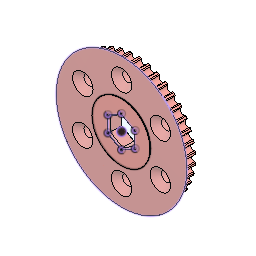
HTD Flanged Pulley Half (Autodesk Fusion 360 design; units mm, degrees)
Autodesk Fusion 360 part; units mm, degrees
sketch "Basic Outline" plane through (0, 0, 0) normal (0, 0, 1) x (1, 0, 0) in component "HTD 5M Pulley"
  circle A0 centre (0, 0) radius 31.2595
  line L0 (0, 0) -> (0, 30.7245) construction
  arc A1 (-1.5246, 30.758) -> (-1.9818, 31.1966) centre (-1.9545, 30.7675) ccw
  arc A2 (-1.5246, 30.758) -> (1.5246, 30.758) centre (0, 30.7245) ccw
  arc A3 (1.9818, 31.1966) -> (1.5246, 30.758) centre (1.9545, 30.7675) ccw
  dimension "d12" = 3.05
  dimension "d19" = 62.519
  dimension "d20" = 29.1995
  dimension "d21" = 0.43
  constraint coincident A0.centre L0.start
  constraint coincident L0.end A2.centre
  constraint tangent A1 A2
  constraint tangent A0 A1
  constraint coincident A0 A1.end
  constraint vertical L0
  constraint tangent A0 A3
  constraint tangent A2 A3
  constraint coincident A0 A3.start
  constraint equal A1 A3
  measures "d12" diameter of A2
  measures "d19" diameter of A0
  measures "d20" distance of A0.centre A2
  measures "d21" radius of A1
extrude "Extrude1" add sketch "Basic Outline" along normal blind 5.5 in component "HTD 5M Pulley"
extrude "Extrude2" cut sketch "Basic Outline" along normal blind 5.5 contours A0 A1 A2 A3 picked at (0, 30.5682) in component "HTD 5M Pulley"
pattern_circular "C-Pattern1" count 40 over 360 about axis through (0, 0, 1.75) along (0, 0, 1) of "Extrude2" in component "HTD 5M Pulley"
sketch "Flange" plane through (0, 0, 5.5) normal (0, 0, 1) x (1, 0, 0) in component "HTD 5M Pulley"
  arc A0 (6.8376, 30.5025) -> (6.3175, 30.1408) centre (6.7436, 30.0829) ccw
  arc A1 (3.3058, 30.6178) -> (6.3175, 30.1408) centre (4.8064, 30.3462) ccw
  arc A2 (3.3058, 30.6178) -> (2.9228, 31.1225) centre (2.8826, 30.6944) ccw
  arc A3 (2.9228, 31.1225) -> (1.9818, 31.1966) centre (0, 0) ccw
  arc A4 (1.9818, 31.1966) -> (1.5246, 30.758) centre (1.9545, 30.7675) ccw
  arc A5 (-1.5246, 30.758) -> (1.5246, 30.758) centre (0, 30.7245) ccw
  arc A6 (-1.5246, 30.758) -> (-1.9818, 31.1966) centre (-1.9545, 30.7675) ccw
  arc A7 (-1.9818, 31.1966) -> (-2.9228, 31.1225) centre (0, 0) ccw
  arc A8 (-2.9228, 31.1225) -> (-3.3058, 30.6178) centre (-2.8826, 30.6944) ccw
  arc A9 (-6.3175, 30.1408) -> (-3.3058, 30.6178) centre (-4.8064, 30.3462) ccw
  arc A10 (-6.3175, 30.1408) -> (-6.8376, 30.5025) centre (-6.7436, 30.0829) ccw
  arc A11 (-6.8376, 30.5025) -> (-7.7555, 30.2821) centre (0, 0) ccw
  arc A12 (-7.7555, 30.2821) -> (-8.0547, 29.7237) centre (-7.6488, 29.8656) ccw
  arc A13 (-10.9548, 28.7815) -> (-8.0547, 29.7237) centre (-9.4944, 29.2207) ccw
  arc A14 (-10.9548, 28.7815) -> (-11.5251, 29.0573) centre (-11.3665, 28.6576) ccw
  arc A15 (-11.5251, 29.0573) -> (-12.3972, 28.6961) centre (0, 0) ccw
  arc A16 (-12.3972, 28.6961) -> (-12.6054, 28.0978) centre (-12.2266, 28.3014) ccw
  arc A17 (-15.3223, 26.7134) -> (-12.6054, 28.0978) centre (-13.9486, 27.3757) ccw
  arc A18 (-15.3223, 26.7134) -> (-15.9287, 26.8967) centre (-15.7096, 26.5267) ccw
  arc A19 (-15.9287, 26.8967) -> (-16.7336, 26.4034) centre (0, 0) ccw
  arc A20 (-16.7336, 26.4034) -> (-16.8457, 25.7799) centre (-16.5034, 26.0402) ccw
  arc A21 (-19.3126, 23.9876) -> (-16.8457, 25.7799) centre (-18.0594, 24.8566) ccw
  arc A22 (-19.3126, 23.9876) -> (-19.9402, 24.0737) centre (-19.6659, 23.7426) ccw
  arc A23 (-19.9402, 24.0737) -> (-20.658, 23.4607) centre (0, 0) ccw
  arc A24 (-20.658, 23.4607) -> (-20.6711, 22.8273) centre (-20.3738, 23.1379) ccw
  arc A25 (-22.8273, 20.6711) -> (-20.6711, 22.8273) centre (-21.7255, 21.7255) ccw
  arc A26 (-22.8273, 20.6711) -> (-23.4607, 20.658) centre (-23.1379, 20.3738) ccw
  arc A27 (-23.4607, 20.658) -> (-24.0737, 19.9402) centre (0, 0) ccw
  arc A28 (-24.0737, 19.9402) -> (-23.9876, 19.3126) centre (-23.7426, 19.6659) ccw
  arc A29 (-25.7799, 16.8457) -> (-23.9876, 19.3126) centre (-24.8566, 18.0594) ccw
  arc A30 (-25.7799, 16.8457) -> (-26.4034, 16.7336) centre (-26.0402, 16.5034) ccw
  arc A31 (-26.4034, 16.7336) -> (-26.8967, 15.9287) centre (0, 0) ccw
  arc A32 (-26.8967, 15.9287) -> (-26.7134, 15.3223) centre (-26.5267, 15.7096) ccw
  arc A33 (-28.0978, 12.6054) -> (-26.7134, 15.3223) centre (-27.3757, 13.9486) ccw
  arc A34 (-28.0978, 12.6054) -> (-28.6961, 12.3972) centre (-28.3014, 12.2266) ccw
  arc A35 (-28.6961, 12.3972) -> (-29.0573, 11.5251) centre (0, 0) ccw
  arc A36 (-29.0573, 11.5251) -> (-28.7815, 10.9548) centre (-28.6576, 11.3665) ccw
  arc A37 (-29.7237, 8.0547) -> (-28.7815, 10.9548) centre (-29.2207, 9.4944) ccw
  arc A38 (-29.7237, 8.0547) -> (-30.2821, 7.7555) centre (-29.8656, 7.6488) ccw
  arc A39 (-30.2821, 7.7555) -> (-30.5025, 6.8376) centre (0, 0) ccw
  arc A40 (-30.5025, 6.8376) -> (-30.1408, 6.3175) centre (-30.0829, 6.7436) ccw
  arc A41 (-30.6178, 3.3058) -> (-30.1408, 6.3175) centre (-30.3462, 4.8064) ccw
  arc A42 (-30.6178, 3.3058) -> (-31.1225, 2.9228) centre (-30.6944, 2.8826) ccw
  arc A43 (-31.1225, 2.9228) -> (-31.1966, 1.9818) centre (0, 0) ccw
  arc A44 (-31.1966, 1.9818) -> (-30.758, 1.5246) centre (-30.7675, 1.9545) ccw
  arc A45 (-30.758, -1.5246) -> (-30.758, 1.5246) centre (-30.7245, 0) ccw
  arc A46 (-30.758, -1.5246) -> (-31.1966, -1.9818) centre (-30.7675, -1.9545) ccw
  arc A47 (-31.1966, -1.9818) -> (-31.1225, -2.9228) centre (0, 0) ccw
  arc A48 (-31.1225, -2.9228) -> (-30.6178, -3.3058) centre (-30.6944, -2.8826) ccw
  arc A49 (-30.1408, -6.3175) -> (-30.6178, -3.3058) centre (-30.3462, -4.8064) ccw
  arc A50 (-30.1408, -6.3175) -> (-30.5025, -6.8376) centre (-30.0829, -6.7436) ccw
  arc A51 (-30.5025, -6.8376) -> (-30.2821, -7.7555) centre (0, 0) ccw
  arc A52 (-30.2821, -7.7555) -> (-29.7237, -8.0547) centre (-29.8656, -7.6488) ccw
  arc A53 (-28.7815, -10.9548) -> (-29.7237, -8.0547) centre (-29.2207, -9.4944) ccw
  arc A54 (-28.7815, -10.9548) -> (-29.0573, -11.5251) centre (-28.6576, -11.3665) ccw
  arc A55 (-29.0573, -11.5251) -> (-28.6961, -12.3972) centre (0, 0) ccw
  arc A56 (-28.6961, -12.3972) -> (-28.0978, -12.6054) centre (-28.3014, -12.2266) ccw
  arc A57 (-26.7134, -15.3223) -> (-28.0978, -12.6054) centre (-27.3757, -13.9486) ccw
  arc A58 (-26.7134, -15.3223) -> (-26.8967, -15.9287) centre (-26.5267, -15.7096) ccw
  arc A59 (-26.8967, -15.9287) -> (-26.4034, -16.7336) centre (0, 0) ccw
  arc A60 (-26.4034, -16.7336) -> (-25.7799, -16.8457) centre (-26.0402, -16.5034) ccw
  arc A61 (-23.9876, -19.3126) -> (-25.7799, -16.8457) centre (-24.8566, -18.0594) ccw
  arc A62 (-23.9876, -19.3126) -> (-24.0737, -19.9402) centre (-23.7426, -19.6659) ccw
  arc A63 (-24.0737, -19.9402) -> (-23.4607, -20.658) centre (0, 0) ccw
  arc A64 (-23.4607, -20.658) -> (-22.8273, -20.6711) centre (-23.1379, -20.3738) ccw
  arc A65 (-20.6711, -22.8273) -> (-22.8273, -20.6711) centre (-21.7255, -21.7255) ccw
  arc A66 (-20.6711, -22.8273) -> (-20.658, -23.4607) centre (-20.3738, -23.1379) ccw
  arc A67 (-20.658, -23.4607) -> (-19.9402, -24.0737) centre (0, 0) ccw
  arc A68 (-19.9402, -24.0737) -> (-19.3126, -23.9876) centre (-19.6659, -23.7426) ccw
  arc A69 (-16.8457, -25.7799) -> (-19.3126, -23.9876) centre (-18.0594, -24.8566) ccw
  arc A70 (-16.8457, -25.7799) -> (-16.7336, -26.4034) centre (-16.5034, -26.0402) ccw
  arc A71 (-16.7336, -26.4034) -> (-15.9287, -26.8967) centre (0, 0) ccw
  arc A72 (-15.9287, -26.8967) -> (-15.3223, -26.7134) centre (-15.7096, -26.5267) ccw
  arc A73 (-12.6054, -28.0978) -> (-15.3223, -26.7134) centre (-13.9486, -27.3757) ccw
  arc A74 (-12.6054, -28.0978) -> (-12.3972, -28.6961) centre (-12.2266, -28.3014) ccw
  arc A75 (-12.3972, -28.6961) -> (-11.5251, -29.0573) centre (0, 0) ccw
  arc A76 (-11.5251, -29.0573) -> (-10.9548, -28.7815) centre (-11.3665, -28.6576) ccw
  arc A77 (-8.0547, -29.7237) -> (-10.9548, -28.7815) centre (-9.4944, -29.2207) ccw
  arc A78 (-8.0547, -29.7237) -> (-7.7555, -30.2821) centre (-7.6488, -29.8656) ccw
  arc A79 (-7.7555, -30.2821) -> (-6.8376, -30.5025) centre (0, 0) ccw
  arc A80 (-6.8376, -30.5025) -> (-6.3175, -30.1408) centre (-6.7436, -30.0829) ccw
  arc A81 (-3.3058, -30.6178) -> (-6.3175, -30.1408) centre (-4.8064, -30.3462) ccw
  arc A82 (-3.3058, -30.6178) -> (-2.9228, -31.1225) centre (-2.8826, -30.6944) ccw
  arc A83 (-2.9228, -31.1225) -> (-1.9818, -31.1966) centre (0, 0) ccw
  arc A84 (-1.9818, -31.1966) -> (-1.5246, -30.758) centre (-1.9545, -30.7675) ccw
  arc A85 (1.5246, -30.758) -> (-1.5246, -30.758) centre (0, -30.7245) ccw
  arc A86 (1.5246, -30.758) -> (1.9818, -31.1966) centre (1.9545, -30.7675) ccw
  arc A87 (1.9818, -31.1966) -> (2.9228, -31.1225) centre (0, 0) ccw
  arc A88 (2.9228, -31.1225) -> (3.3058, -30.6178) centre (2.8826, -30.6944) ccw
  arc A89 (6.3175, -30.1408) -> (3.3058, -30.6178) centre (4.8064, -30.3462) ccw
  arc A90 (6.3175, -30.1408) -> (6.8376, -30.5025) centre (6.7436, -30.0829) ccw
  arc A91 (6.8376, -30.5025) -> (7.7555, -30.2821) centre (0, 0) ccw
  arc A92 (7.7555, -30.2821) -> (8.0547, -29.7237) centre (7.6488, -29.8656) ccw
  arc A93 (10.9548, -28.7815) -> (8.0547, -29.7237) centre (9.4944, -29.2207) ccw
  arc A94 (10.9548, -28.7815) -> (11.5251, -29.0573) centre (11.3665, -28.6576) ccw
  arc A95 (11.5251, -29.0573) -> (12.3972, -28.6961) centre (0, 0) ccw
  arc A96 (12.3972, -28.6961) -> (12.6054, -28.0978) centre (12.2266, -28.3014) ccw
  arc A97 (15.3223, -26.7134) -> (12.6054, -28.0978) centre (13.9486, -27.3757) ccw
  arc A98 (15.3223, -26.7134) -> (15.9287, -26.8967) centre (15.7096, -26.5267) ccw
  arc A99 (15.9287, -26.8967) -> (16.7336, -26.4034) centre (0, 0) ccw
  arc A100 (16.7336, -26.4034) -> (16.8457, -25.7799) centre (16.5034, -26.0402) ccw
  arc A101 (19.3126, -23.9876) -> (16.8457, -25.7799) centre (18.0594, -24.8566) ccw
  arc A102 (19.3126, -23.9876) -> (19.9402, -24.0737) centre (19.6659, -23.7426) ccw
  arc A103 (19.9402, -24.0737) -> (20.658, -23.4607) centre (0, 0) ccw
  arc A104 (20.658, -23.4607) -> (20.6711, -22.8273) centre (20.3738, -23.1379) ccw
  arc A105 (22.8273, -20.6711) -> (20.6711, -22.8273) centre (21.7255, -21.7255) ccw
  arc A106 (22.8273, -20.6711) -> (23.4607, -20.658) centre (23.1379, -20.3738) ccw
  arc A107 (23.4607, -20.658) -> (24.0737, -19.9402) centre (0, 0) ccw
  arc A108 (24.0737, -19.9402) -> (23.9876, -19.3126) centre (23.7426, -19.6659) ccw
  arc A109 (25.7799, -16.8457) -> (23.9876, -19.3126) centre (24.8566, -18.0594) ccw
  arc A110 (25.7799, -16.8457) -> (26.4034, -16.7336) centre (26.0402, -16.5034) ccw
  arc A111 (26.4034, -16.7336) -> (26.8967, -15.9287) centre (0, 0) ccw
  arc A112 (26.8967, -15.9287) -> (26.7134, -15.3223) centre (26.5267, -15.7096) ccw
  arc A113 (28.0978, -12.6054) -> (26.7134, -15.3223) centre (27.3757, -13.9486) ccw
  arc A114 (28.0978, -12.6054) -> (28.6961, -12.3972) centre (28.3014, -12.2266) ccw
  arc A115 (28.6961, -12.3972) -> (29.0573, -11.5251) centre (0, 0) ccw
  arc A116 (29.0573, -11.5251) -> (28.7815, -10.9548) centre (28.6576, -11.3665) ccw
  arc A117 (29.7237, -8.0547) -> (28.7815, -10.9548) centre (29.2207, -9.4944) ccw
  arc A118 (29.7237, -8.0547) -> (30.2821, -7.7555) centre (29.8656, -7.6488) ccw
  arc A119 (30.2821, -7.7555) -> (30.5025, -6.8376) centre (0, 0) ccw
  arc A120 (30.5025, -6.8376) -> (30.1408, -6.3175) centre (30.0829, -6.7436) ccw
  arc A121 (30.6178, -3.3058) -> (30.1408, -6.3175) centre (30.3462, -4.8064) ccw
  arc A122 (30.6178, -3.3058) -> (31.1225, -2.9228) centre (30.6944, -2.8826) ccw
  arc A123 (31.1225, -2.9228) -> (31.1966, -1.9818) centre (0, 0) ccw
  arc A124 (31.1966, -1.9818) -> (30.758, -1.5246) centre (30.7675, -1.9545) ccw
  arc A125 (30.758, 1.5246) -> (30.758, -1.5246) centre (30.7245, 0) ccw
  arc A126 (30.758, 1.5246) -> (31.1966, 1.9818) centre (30.7675, 1.9545) ccw
  arc A127 (31.1966, 1.9818) -> (31.1225, 2.9228) centre (0, 0) ccw
  arc A128 (31.1225, 2.9228) -> (30.6178, 3.3058) centre (30.6944, 2.8826) ccw
  arc A129 (30.1408, 6.3175) -> (30.6178, 3.3058) centre (30.3462, 4.8064) ccw
  arc A130 (30.1408, 6.3175) -> (30.5025, 6.8376) centre (30.0829, 6.7436) ccw
  arc A131 (30.5025, 6.8376) -> (30.2821, 7.7555) centre (0, 0) ccw
  arc A132 (30.2821, 7.7555) -> (29.7237, 8.0547) centre (29.8656, 7.6488) ccw
  arc A133 (28.7815, 10.9548) -> (29.7237, 8.0547) centre (29.2207, 9.4944) ccw
  arc A134 (28.7815, 10.9548) -> (29.0573, 11.5251) centre (28.6576, 11.3665) ccw
  arc A135 (29.0573, 11.5251) -> (28.6961, 12.3972) centre (0, 0) ccw
  arc A136 (28.6961, 12.3972) -> (28.0978, 12.6054) centre (28.3014, 12.2266) ccw
  arc A137 (26.7134, 15.3223) -> (28.0978, 12.6054) centre (27.3757, 13.9486) ccw
  arc A138 (26.7134, 15.3223) -> (26.8967, 15.9287) centre (26.5267, 15.7096) ccw
  arc A139 (26.8967, 15.9287) -> (26.4034, 16.7336) centre (0, 0) ccw
  arc A140 (26.4034, 16.7336) -> (25.7799, 16.8457) centre (26.0402, 16.5034) ccw
  arc A141 (23.9876, 19.3126) -> (25.7799, 16.8457) centre (24.8566, 18.0594) ccw
  arc A142 (23.9876, 19.3126) -> (24.0737, 19.9402) centre (23.7426, 19.6659) ccw
  arc A143 (24.0737, 19.9402) -> (23.4607, 20.658) centre (0, 0) ccw
  arc A144 (23.4607, 20.658) -> (22.8273, 20.6711) centre (23.1379, 20.3738) ccw
  arc A145 (20.6711, 22.8273) -> (22.8273, 20.6711) centre (21.7255, 21.7255) ccw
  arc A146 (20.6711, 22.8273) -> (20.658, 23.4607) centre (20.3738, 23.1379) ccw
  arc A147 (20.658, 23.4607) -> (19.9402, 24.0737) centre (0, 0) ccw
  arc A148 (19.9402, 24.0737) -> (19.3126, 23.9876) centre (19.6659, 23.7426) ccw
  arc A149 (16.8457, 25.7799) -> (19.3126, 23.9876) centre (18.0594, 24.8566) ccw
  arc A150 (16.8457, 25.7799) -> (16.7336, 26.4034) centre (16.5034, 26.0402) ccw
  arc A151 (16.7336, 26.4034) -> (15.9287, 26.8967) centre (0, 0) ccw
  arc A152 (15.9287, 26.8967) -> (15.3223, 26.7134) centre (15.7096, 26.5267) ccw
  arc A153 (12.6054, 28.0978) -> (15.3223, 26.7134) centre (13.9486, 27.3757) ccw
  arc A154 (12.6054, 28.0978) -> (12.3972, 28.6961) centre (12.2266, 28.3014) ccw
  arc A155 (12.3972, 28.6961) -> (11.5251, 29.0573) centre (0, 0) ccw
  arc A156 (11.5251, 29.0573) -> (10.9548, 28.7815) centre (11.3665, 28.6576) ccw
  arc A157 (8.0547, 29.7237) -> (10.9548, 28.7815) centre (9.4944, 29.2207) ccw
  arc A158 (8.0547, 29.7237) -> (7.7555, 30.2821) centre (7.6488, 29.8656) ccw
  arc A159 (7.7555, 30.2821) -> (6.8376, 30.5025) centre (0, 0) ccw
  circle A160 centre (0, 0) radius 31.2595 construction
  circle A161 centre (0, 0) radius 33.7595
  circle A162 centre (0, 0) radius 83.7595
  dimension "d58" = 2.5
  dimension "d59" = 50
  constraint concentric A160 A161
  constraint concentric A3 A162
  measures "d58" distance of A160 A161
  measures "d59" distance of A161 A162
extrude "Extrude3" add sketch "Basic Outline" along normal blind 1.45 draft 60 from surface at 5.5 in component "HTD 5M Pulley"
extrude "Extrude4" cut sketch "Flange" along normal through all contours A162 in component "HTD 5M Pulley"
sketch "Axle and Bolts" plane through (0, 0, 6.95) normal (0, 0, 1) x (1, 0, 0) in component "HTD 5M Pulley"
  circle A0 centre (0, 0) radius 33.7595
  circle A1 centre (0, 0) radius 31.2595 construction
  line L0 (0, 0) -> (0, 30.7245) construction
  line L1 (0, 7.4057) -> (-6.4135, 3.7028)
  line L2 (-6.4135, 3.7028) -> (-6.4135, -3.7028)
  line L3 (-6.4135, -3.7028) -> (0, -7.4057)
  line L4 (0, -7.4057) -> (6.4135, -3.7028)
  line L5 (6.4135, -3.7028) -> (6.4135, 3.7028)
  line L6 (6.4135, 3.7028) -> (0, 7.4057)
  point P0 (0, 23.1297)
  dimension "d60" = 6.4135
  dimension "d63" = 23.1297
  constraint coincident A0.centre A1.centre
  constraint coincident L0 L1.start
  constraint coincident L0 P0
  measures "d60" distance of A0.centre L6
  measures "d63" distance of A0.centre P0
extrude "Extrude6" cut sketch "Axle and Bolts" against normal through all contours L1 L2 L3 L4 L5 L6 in component "HTD 5M Pulley"
chamfer "Chamfer1" distance 0.6 angle 45 12 edges at (-3.2068, 5.5543, 6.95) (3.2068, 5.5543, 6.95) (6.4135, 0, 6.95) (3.2067, -5.5543, 6.95) (-3.2068, -5.5543, 6.95) (-6.4135, 0, 6.95) (-6.4135, 0, 0) (-3.2068, 5.5543, 0) (-3.2068, -5.5543, 0) (3.2068, 5.5543, 0) (6.4135, 0, 0) (3.2067, -5.5543, 0) in component "HTD 5M Pulley"
sketch "Hub" plane through (0, 0, 6.95) normal (0, 0, 1) x (1, 0, 0) in component "HTD 5M Pulley"
  circle A0 centre (0, 0) radius 33.7595
  line L0 (7.0135, -4.0492) -> (0, -8.0985)
  line L1 (0, -8.0985) -> (-7.0135, -4.0492)
  line L2 (-7.0135, -4.0492) -> (-7.0135, 4.0492)
  line L3 (-7.0135, 4.0492) -> (0, 8.0985)
  line L4 (0, 8.0985) -> (7.0135, 4.0492)
  line L5 (7.0135, 4.0492) -> (7.0135, -4.0492)
  circle A1 centre (0, 0) radius 15
  dimension "d64" = 30
  constraint concentric A0 A1
  measures "d64" diameter of A1
extrude "Extrude7" add sketch "Hub" along normal blind 0.3 contours A1 in component "HTD 5M Pulley"
hole "Hole1" at (0, 23.1297, 6.95) direction (0, 0, -1) diameter 5.105 end through all countersink diameter 9.779 countersink angle 82 in component "HTD 5M Pulley"
pattern_circular "C-Pattern2" count 6 over 360 about axis through (0, 0, 1.75) along (0, 0, 1) of "Hole1" in component "HTD 5M Pulley"
move_face "OffsetFaces1" offset -0.3 6 faces at (3.9374, 25.0259, 6.3526) (24.207, 10.2767, 6.3526) (21.0034, -15.8255, 6.3526) (1.5966, -27.1978, 6.3526) (-17.8459, -7.7802, 6.3526) (-22.216, 15.3495, 6.3526) in component "HTD 5M Pulley"
component "HTD 5M Pulley" placed x (1, 0, 0) y (0, 1, 0) z (0, 0, 1) at (0, 0, 0)
equation "NUM_TEETH = 40" comment "Number of teeth in the pulley"
equation "TOOTH_PITCH = 5 mm" comment "Belt pitch (ie: 5mm=HTD5)"
equation "zOutsideDia = 2 * ( ( NUM_TEETH * TOOTH_PITCH ) / ( PI * 2 ) - zPitchLineOffset )"
equation "zPitchLineOffset = 0.5715 mm"
equation "zToothDia = 2.06 mm"
equation "zMinorDia = zOutsideDia - 2 * zToothDia"
equation "zToothWidth = 3.05 mm"
equation "zToothRootDia = 0.86 mm"
equation "d12 = zToothWidth"
equation "d17 = TOOTH_WIDTH / 2"
equation "d19 = zOutsideDia"
equation "d20 = $MinorDia / 2"
equation "d21 = zToothRootDia / 2"
equation "d22 = d17"
equation "d24 = NUM_TEETH"
equation "TOOTH_WIDTH = 11 mm" comment "Width of the toothed part of the pulley"
equation "TOTAL_WIDTH = 14.5 mm" comment "Total width of the pulley at the hub"
equation "PRINTER_LAYER_HEIGHT = 0.3 mm" comment "Layer height of printer (typically 0.2mm or 0.3mm)"
equation "HUB_OFFSET = if(PRINTER_LAYER_HEIGHT >= 0.3 mm; PRINTER_LAYER_HEIGHT; PRINTER_LAYER_HEIGHT * 2)" comment "Distant hub projects above rim (so rim won't scrape when pulley rotates)"
equation "FLANGE_ANGLE = 60 deg" comment "Typically 60 if printing with a hub offset, 80 otherwise"
equation "HEX_SHAFT_DIAMETER = 0.505 in" comment "Hex shaft diameter + tolerance"
equation "d34 = ( TOTAL_WIDTH - TOOTH_WIDTH ) / 2 - HUB_OFFSET"
equation "d35 = FLANGE_ANGLE"
equation "FLANGE_MAX_HEIGHT = 2.5 mm" comment "Max height of the flange"
equation "HUB_DIAMETER = 30 mm" comment "Diameter of the raised hub"
equation "NUM_BOLTS = 6" comment "Number of mounting bolts (edit feature to change type)"
equation "d52 = NUM_BOLTS"
equation "d54 = PRINTER_LAYER_HEIGHT * 2"
equation "d55 = -PRINTER_LAYER_HEIGHT"
equation "d58 = FLANGE_MAX_HEIGHT"
equation "d60 = HEX_SHAFT_DIAMETER / 2"
equation "BOLT_RADIUS = ( zOutsideDia + HUB_DIAMETER ) / 4" comment "Radius of the bolt circle (default is halfway between hub and rim)"
equation "d63 = BOLT_RADIUS"
equation "d64 = HUB_DIAMETER"
equation "d65 = HUB_OFFSET"
